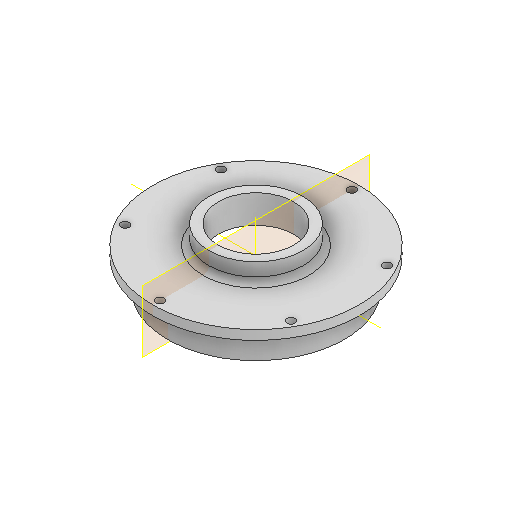
# Autodesk Inventor part: Deckel Stempel
Saved by Autodesk Inventor 2023 (Build 270158000, 158)
## iProperties
Created: 2022-11-23
Part Number: Deckel Stempel
Material: Generisch
Document SubType Name: Modeling
Designer: schil
Density: 1 g/cm^3
Appearance: Vorgabe
Author: schil
Autodesk Inventor part; units mm, degrees
ref_plane "XZ Plane" through (0, 0, 0) normal (0, 1, 0) x (-1, 0, 0)
ref_plane "XY Plane" through (0, 0, 0) normal (0, 0, 1) x (1, 0, 0)
sketch "Skizze1" plane through (0, 0, 0) normal (1, 0, 0) x (0, 1, 0)
  line L0 (15, -20) -> (5, -20)
  line L1 (5, -20) -> (5, -25)
  line L2 (5, -25) -> (15, -25)
  line L3 (15, -25) -> (15, -20)
  line L4 (5, -20) -> (0, -20)
  line L5 (0, -20) -> (0, -55)
  line L6 (0, -55) -> (5, -55)
  line L7 (5, -55) -> (5, -20)
  line L8 (0, -47) -> (-15, -47)
  line L9 (-15, -47) -> (-15, -42)
  line L10 (-15, -42) -> (0, -42)
  line L11 (0, -42) -> (0, -47)
  line L12 (0, -42) -> (-2, -42)
  line L13 (-2, -42) -> (-2, -37.5)
  line L14 (-2, -37.5) -> (0, -37.5)
  line L15 (0, -37.5) -> (0, -42)
  line L16 (-21, 0) -> (21, 0) projected
  line L17 (0, -66) -> (0, 11) projected
  point P0 (0, 0)
  point P1 (10, -25)
  point P2 (10, -20)
  point P3 (0, -44.5)
  point P4 (2.5, -55)
  point P5 (-7.5, -47)
  point P6 (0, -37.5)
  point P7 (-2, -42)
  point P8 (5, -25)
  dimension "d0" = 5
  dimension "d1" = 5
  dimension "d2" = 35
  dimension "d3" = 10
  dimension "d4" = 8
  dimension "d5" = 5
  dimension "d6" = 15
  dimension "d7" = 20
  dimension "d8" = 2
  dimension "d9" = 4.5
  dimension "d10" = 0
  constraints: 32 end point, 8 parallel, 5 midpoint, 4 horizontal, 4 perpendicular, 1 point on line
  measures "d0" distance of point (10, -25) point (10, -20)
  measures "d1" distance from line of point (0, -44.5) L7
  measures "d2" distance from line of point (2.5, -55) L0
  measures "d3" distance of L1.end L2.end
  measures "d4" distance from line of point (2.5, -55) L8
  measures "d5" distance from line of point (-7.5, -47) L10
  measures "d6" distance of L8.start L8.end
  measures "d7" distance from line of L16 L0.start
  measures "d8" distance of L13.end L14.end
  measures "d9" distance of L12.end L13.end
  measures "d10" distance between parallel lines of L17 L5
revolve "Umdrehung1" add sketch "Skizze1" angle 360 about axis through (0, -10, 0) along (0, 1, 0)
fillet "Rundung1" radius 3 1 edges at (0, 5, 25)
fillet "Rundung2" radius 2 1 edges at (0, -2, 42)
sketch "Skizze2" plane through (0, 5, 0) normal (0, 1, 0) x (1, 0, 0)
  line L0 (-77, 0) -> (77, 0) projected
  line L1 (0, 77) -> (0, -77) projected
  circle A0 centre (0, 0) radius 51
  circle A1 centre (0, 0) radius 55 projected
  point P0 (0, -51)
  point P1 (44.1673, -25.5)
  point P2 (44.1673, 25.5)
  point P3 (0, 51)
  point P4 (-44.1673, 25.5)
  point P5 (-44.1673, -25.5)
  dimension "d14" = 4
  dimension "d17" = 360
  constraints: 1 coincident, 1 point on line, 1 vertical alignment, 9 other
hole "Bohrung1" at (0, 5, 51) at (44.1673, 5, 25.5) at (44.1673, 5, -25.5) at (0, 5, -51) at (-44.1673, 5, -25.5) at (-44.1673, 5, 25.5) direction (0, -1, 0) diameter 4.5 depth 11.8 tip angle 118
